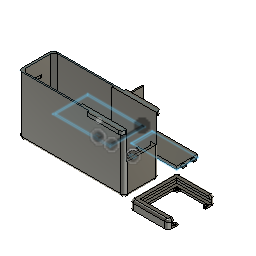
autodoorlock_main_casing v4 (Autodesk Fusion 360 design; units mm, degrees)
Autodesk Fusion 360 part; units mm, degrees
sketch "Sketch1" plane through (0, 0, 0) normal (0, 0, 1) x (1, 0, 0)
  line L0 (-75, 25) -> (75, 25)
  line L1 (75, 25) -> (75, -25)
  line L2 (75, -25) -> (-75, -25)
  line L3 (-75, -25) -> (-75, 25)
  line L4 (16.5, -10.5) -> (58.5, -10.5)
  line L5 (58.5, -10.5) -> (58.5, 10.5)
  line L6 (58.5, 10.5) -> (16.5, 10.5)
  line L7 (16.5, 10.5) -> (16.5, -10.5)
  line L8 (16.5, -10.5) -> (58.5, 10.5) construction
  line L9 (58.5, -10.5) -> (16.5, 10.5) construction
  line L10 (9.5, 10.5) -> (9.5, -10.5065)
  line L11 (16.5, -10.5065) -> (16.5, 10.5)
  line L12 (65.5, 10.5) -> (65.5, -10.5)
  line L13 (58.5, -10.5) -> (58.5, 10.5)
  line L14 (9.5, 10.5) -> (6.5, 10.5)
  line L15 (6.5, 10.5) -> (6.5, -10.5)
  line L16 (6.5, -10.5) -> (9.5, -10.5)
  line L17 (9.5, -10.5) -> (9.5, 10.5)
  line L18 (65.5, 10.5) -> (68.5, 10.5)
  line L19 (68.5, 10.5) -> (68.5, -10.5)
  line L20 (68.5, -10.5) -> (65.5, -10.5)
  line L21 (65.5, -10.5) -> (65.5, 10.5)
  point P0 (37.5, 0)
  dimension "d1" = 150
  dimension "d2" = 50
  dimension "d3" = 42
  dimension "d4" = 21
  dimension "d5" = 7
  dimension "d6" = 7
  dimension "d7" = 21
  dimension "d8" = 3
  dimension "d9" = 21
  dimension "d10" = 3
  dimension "d11" = 21
  constraint horizontal L0
  constraint vertical L1
  constraint horizontal L2
  constraint vertical L3
  constraint horizontal L4
  constraint perpendicular L4 L5
  constraint parallel L4 L6
  constraint parallel L5 L7
  constraint coincident L8 P0
  constraint coincident L9 P0
  constraint vertical L10
  constraint vertical L11
  constraint vertical L12
  constraint vertical L13
  constraint horizontal L14
  constraint vertical L15
  constraint horizontal L16
  constraint vertical L17
  constraint horizontal L18
  constraint vertical L19
  constraint horizontal L20
  constraint vertical L21
  measures "d1" distance of L0.start L0.end
  measures "d2" distance of L0.start L2.end
  measures "d3" distance of L5.end L6.end
  measures "d4" distance of L4.end L5.end
  measures "d5" distance of L6.end L10.start
  measures "d6" distance of L5.end L12.start
  measures "d7" distance of L5.end L4.end
  measures "d8" distance of L10.start L14.end
  measures "d9" distance of L10.start L16.end
  measures "d10" distance of L12.start L18.end
  measures "d11" distance of L12.start L12.end
extrude "Extrude1" add sketch "Sketch1" along normal blind 5 makes body 1
extrude "Extrude2" add sketch "Sketch1" along normal blind 40 contours L10 L14 L15 L16 L17 | L12 L18 L19 L20 L21 bodies 1
sketch "Sketch2" plane through (9.5, 0, 0) normal (1, 0, 0) x (0, 1, 0)
  line L0 (-10.5, 5) -> (10.5, 5)
  line L1 (10.5, 5) -> (10.5, 40)
  line L2 (10.5, 40) -> (-10.5, 40)
  line L3 (-10.5, 40) -> (-10.5, 5)
  line L4 (-10.5, 40) -> (10.5, 40)
  line L5 (10.5, 40) -> (10.5, 35)
  line L6 (10.5, 35) -> (-10.5, 35)
  line L7 (-10.5, 35) -> (-10.5, 40)
  dimension "d16" = 5
  constraint horizontal L4
  constraint vertical L5
  constraint horizontal L6
  constraint vertical L7
  constraint coincident L2.end L3.start
  measures "d16" distance of L2.end L6.end
extrude "Extrude3" add sketch "Sketch2" along normal blind 6 contours L1 L2 L3 L4 L5 L6 L7 bodies 1
sketch "Sketch3" plane through (65.5, 0, 0) normal (-1, 0, 0) x (0, -1, 0)
  line L0 (-10.5, 5) -> (10.5, 5)
  line L1 (10.5, 5) -> (10.5, 40)
  line L2 (10.5, 40) -> (-10.5, 40)
  line L3 (-10.5, 40) -> (-10.5, 5)
  line L4 (-10.5, 40) -> (10.5, 40)
  line L5 (10.5, 40) -> (10.5, 35)
  line L6 (10.5, 35) -> (-10.5, 35)
  line L7 (-10.5, 35) -> (-10.5, 40)
  dimension "d19" = 5
  constraint horizontal L4
  constraint vertical L5
  constraint horizontal L6
  constraint vertical L7
  constraint coincident L2.end L3.start
  measures "d19" distance of L2.end L6.end
extrude "Extrude4" add sketch "Sketch3" along normal blind 6 contours L1 L2 L3 L4 L5 L6 L7 bodies 1
chamfer "Chamfer1" distance 3 angle 45 1 edges at (65.5, 0, 5) on bodies 1
chamfer "Chamfer2" distance 3 angle 45 1 edges at (9.5, 0, 5) on bodies 1
chamfer "Chamfer3" distance 3 angle 45 1 edges at (68.5, 0, 5) on bodies 1
chamfer "Chamfer4" distance 3 angle 45 1 edges at (6.5, 0, 5) on bodies 1
chamfer "Chamfer5" distance 3 angle 45 1 edges at (67, -10.5, 5) on bodies 1
chamfer "Chamfer6" distance 3 angle 45 1 edges at (67, 10.5, 5) on bodies 1
chamfer "Chamfer7" distance 3 angle 45 1 edges at (8, 10.5, 5) on bodies 1
chamfer "Chamfer8" distance 3 angle 45 1 edges at (8, -10.5, 5) on bodies 1
sketch "Sketch4" plane through (0, 0, 40) normal (0, 0, 1) x (-1, 0, 0)
  line L0 (-15.5, -10.5) -> (-6.5, -10.5)
  line L1 (-6.5, -10.5) -> (-6.5, 10.5)
  line L2 (-6.5, 10.5) -> (-15.5, 10.5)
  line L3 (-15.5, 10.5) -> (-15.5, -10.5)
  circle A0 centre (-13.25, 5.25) radius 2.5
  circle A1 centre (-13.25, -5.25) radius 2.5
  dimension "d30" = 5
  dimension "d31" = 5
  measures "d30" diameter of A0
  measures "d31" diameter of A1
extrude "Extrude5" cut sketch "Sketch4" against normal blind 7 contours L3 A1 | L3 A0 picked at (-13.4213, -4.5833) picked at (-12.8787, 5.7617) bodies 1
sketch "Sketch5" plane through (0, 0, 40) normal (0, 0, 1) x (-1, 0, 0)
  line L0 (-59.5, 10.5) -> (-68.5, 10.5)
  line L1 (-68.5, 10.5) -> (-68.5, -10.5)
  line L2 (-68.5, -10.5) -> (-59.5, -10.5)
  line L3 (-59.5, -10.5) -> (-59.5, 10.5)
  circle A0 centre (-61.75, 5.25) radius 2.5
  circle A1 centre (-61.75, -5.25) radius 2.5
  dimension "d34" = 5
  dimension "d35" = 5
  measures "d34" diameter of A0
  measures "d35" diameter of A1
extrude "Extrude6" cut sketch "Sketch5" against normal blind 7 contours L3 A0 | L3 A1 picked at (-61.1713, 5.0046) picked at (-61.1713, -5.4954) bodies 1
extrude "Extrude7" add sketch "Sketch1" along normal blind 5 contours L4 L5 L6 L7 L11 L13 bodies 1
sketch "Sketch6" plane through (0, 0, 35) normal (0, 0, -1) x (1, 0, 0)
  arc A0 (15.5, -4.1603) -> (15.5, -6.3397) centre (13.25, -5.25) ccw
  line L0 (15.5, -4.1603) -> (15.5, 4.1603)
  arc A1 (15.5, 6.3397) -> (15.5, 4.1603) centre (13.25, 5.25) ccw
  line L1 (15.5, 6.3397) -> (15.5, 10.5)
  line L2 (15.5, 10.5) -> (9.5, 10.5)
  line L3 (9.5, 10.5) -> (9.5, -10.5)
  line L4 (9.5, -10.5) -> (15.5, -10.5)
  line L5 (15.5, -10.5) -> (15.5, -6.3397)
  line L6 (15.5, 1.5) -> (9.5, 1.5)
  line L7 (9.5, 1.5) -> (9.5, -1.5)
  line L8 (9.5, -1.5) -> (15.5, -1.5)
  line L9 (15.5, -1.5) -> (15.5, 1.5)
  line L10 (15.5, 1.5) -> (9.5, -1.5) construction
  line L11 (9.5, 1.5) -> (15.5, -1.5) construction
  point P0 (12.5, 0)
  constraint horizontal L6
  constraint perpendicular L6 L7
  constraint parallel L6 L8
  constraint parallel L7 L9
  constraint coincident L10 P0
  constraint coincident L11 P0
  constraint coincident L0 L6.start
delete_face "DeleteFace1" 1 faces at (11.5, -3.5, 6) on bodies 1
delete_face "DeleteFace2" 1 faces at (63.5, -3.5, 6) on bodies 1
sketch "Sketch7" plane through (0, 0, 35) normal (0, 0, -1) x (1, 0, 0)
  arc A0 (59.5, 4.1603) -> (59.5, 6.3397) centre (61.75, 5.25) ccw
  line L0 (59.5, 4.1603) -> (59.5, -4.1603)
  arc A1 (59.5, -6.3397) -> (59.5, -4.1603) centre (61.75, -5.25) ccw
  line L1 (59.5, -6.3397) -> (59.5, -10.5)
  line L2 (59.5, -10.5) -> (65.5, -10.5)
  line L3 (65.5, -10.5) -> (65.5, 10.5)
  line L4 (65.5, 10.5) -> (59.5, 10.5)
  line L5 (59.5, 10.5) -> (59.5, 6.3397)
  line L6 (59.5, 1.5) -> (65.5, 1.5)
  line L7 (65.5, 1.5) -> (65.5, -1.5)
  line L8 (65.5, -1.5) -> (59.5, -1.5)
  line L9 (59.5, -1.5) -> (59.5, 1.5)
  line L10 (59.5, 1.5) -> (65.5, -1.5) construction
  line L11 (65.5, 1.5) -> (59.5, -1.5) construction
  point P0 (62.5, 0)
  dimension "d42" = 3
  constraint horizontal L6
  constraint perpendicular L6 L7
  constraint parallel L6 L8
  constraint parallel L7 L9
  constraint coincident L10 P0
  constraint coincident L11 P0
  measures "d42" distance of L6.end L7.end
extrude "Extrude9" add sketch "Sketch7" along normal blind 30 contours L0 L3 L6 L7 L8 L9 bodies 1
chamfer "Chamfer9" distance 3 angle 45 2 edges at (65.5, 7.5, 5) (62.5, 1.5, 5) on bodies 1
chamfer "Chamfer10" distance 3 angle 45 2 edges at (65.5, -7.5, 5) (62.5, -1.5, 5) on bodies 1
chamfer "Chamfer14" distance 3 angle 45 1 edges at (59.5, 0, 5) on bodies 1
chamfer "Chamfer15" distance 3 angle 45 1 edges at (9.5, 0, 5) on bodies 1
extrude "Extrude10" add sketch "Sketch6" along normal blind 5 contours L0 L3 L6 L7 L8 L9 bodies 1
chamfer "Chamfer16" distance 5 angle 45 1 edges at (15.5, 0, 30) on bodies 1
sketch "Sketch8" plane through (-75, 0, 0) normal (-1, 0, 0) x (0, -1, 0)
  line L0 (-25, 0) -> (25, 0)
  line L1 (25, 0) -> (25, 5)
  line L2 (25, 5) -> (-25, 5)
  line L3 (-25, 5) -> (-25, 0)
  line L4 (-15, 0) -> (15, 0)
  line L5 (15, 0) -> (15, 5)
  line L6 (15, 5) -> (-15, 5)
  line L7 (-15, 5) -> (-15, 0)
  line L8 (-15, 0) -> (15, 5) construction
  line L9 (15, 0) -> (-15, 5) construction
  point P0 (0, 2.5)
  dimension "d55" = 30
  constraint horizontal L4
  constraint perpendicular L4 L5
  constraint parallel L4 L6
  constraint parallel L5 L7
  constraint coincident L8 P0
  constraint coincident L9 P0
  measures "d55" distance of L5.end L6.end
extrude "Extrude11" cut sketch "Sketch8" against normal blind 65 contours L0 L2 L4 L5 L6 L7 bodies 1
sketch "Sketch9" plane through (0, 0, 5) normal (0, 0, 1) x (-1, 0, 0)
  line L0 (10, 15) -> (75, 15)
  line L1 (75, 15) -> (75, 25)
  line L2 (75, 25) -> (-75, 25)
  line L3 (-75, 25) -> (-75, -25)
  line L4 (-75, -25) -> (75, -25)
  line L5 (75, -25) -> (75, -15)
  line L6 (75, -15) -> (10, -15)
  line L7 (10, -15) -> (10, 15)
  line L8 (-12.5, 13.5) -> (-3.5, 13.5)
  line L9 (-3.5, 13.5) -> (-3.5, -13.5)
  line L10 (-3.5, -13.5) -> (-12.5, -13.5)
  line L11 (-12.5, -13.5) -> (-12.5, 13.5)
  line L12 (-56.5, -4.5) -> (-62.5, -4.5)
  line L13 (-62.5, -4.5) -> (-62.5, -13.5)
  line L14 (-62.5, -13.5) -> (-71.5, -13.5)
  line L15 (-71.5, -13.5) -> (-71.5, 13.5)
  line L16 (-71.5, 13.5) -> (-62.5, 13.5)
  line L17 (-62.5, 13.5) -> (-62.5, 4.5)
  line L18 (-62.5, 4.5) -> (-56.5, 4.5)
  line L19 (-56.5, 4.5) -> (-56.5, -4.5)
  line L20 (10, -15) -> (5, -15)
  line L21 (5, -15) -> (5, 15)
  line L22 (5, 15) -> (10, 15)
  line L23 (10, 15) -> (10, -15)
  dimension "d58" = 5
  dimension "d59" = 30
  constraint horizontal L20
  constraint vertical L21
  constraint horizontal L22
  constraint vertical L23
  constraint coincident L6.end L7.start
  measures "d58" distance of L6.end L20.end
  measures "d59" distance of L6.end L0.start
sketch "Sketch10" plane through (0, 0, 5) normal (0, 0, 1) x (-1, 0, 0)
  line L0 (5, 15) -> (75, 15)
  line L1 (75, 15) -> (75, 17)
  line L2 (75, 17) -> (5, 17)
  line L3 (5, 17) -> (5, 15)
  line L4 (5, -15) -> (75, -15)
  line L5 (75, -15) -> (75, -17)
  line L6 (75, -17) -> (5, -17)
  line L7 (5, -17) -> (5, -15)
  point P0 (5, 15)
  point P1 (5, -15)
  dimension "d60" = 2
  dimension "d61" = 2
  constraint horizontal L0
  constraint vertical L1
  constraint horizontal L2
  constraint vertical L3
  constraint coincident P0 L0.start
  constraint horizontal L4
  constraint vertical L5
  constraint horizontal L6
  constraint vertical L7
  constraint coincident P1 L4.start
  measures "d60" distance of P0 L2.end
  measures "d61" distance of P1 L6.end
extrude "Extrude12" add sketch "Sketch10" sketch "Sketch9" along normal blind 20 of sketch 2 contours L7 L20 L21 L22 L23 bodies 1
sketch "Sketch11" plane through (0, 0, 25) normal (0, 0, 1) x (-1, 0, 0)
  line L0 (5, -17) -> (75, -17)
  line L1 (75, -17) -> (75, -15)
  line L2 (75, -15) -> (10, -15)
  line L3 (10, -15) -> (10, 15)
  line L4 (10, 15) -> (75, 15)
  line L5 (75, 15) -> (75, 17)
  line L6 (75, 17) -> (5, 17)
  line L7 (5, 17) -> (5, -17)
  line L8 (5, -17) -> (75, -17)
  line L9 (75, -17) -> (75, 17)
  line L10 (75, 17) -> (5, 17)
  line L11 (5, 17) -> (5, -17)
  constraint horizontal L8
  constraint vertical L9
  constraint horizontal L10
  constraint vertical L11
  constraint coincident L5.end L6.start
  constraint coincident L0.start L7.end
extrude "Extrude13" add sketch "Sketch11" along normal blind 3 bodies 1
sketch "Sketch12" plane through (0, -15, 0) normal (0, 1, 0) x (-1, 0, 0)
  line L0 (75, 0) -> (75, 25)
  line L1 (75, 25) -> (10, 25)
  line L2 (10, 25) -> (10, 0)
  line L3 (10, 0) -> (75, 0)
  line L4 (10, 20.5612) -> (13, 20.5612)
  line L5 (13, 20.5612) -> (13, 5.5612)
  line L6 (13, 5.5612) -> (10, 5.5612)
  line L7 (10, 5.5612) -> (10, 20.5612)
  dimension "d66" = 3
  dimension "d67" = 15
  constraint horizontal L4
  constraint vertical L5
  constraint horizontal L6
  constraint vertical L7
  constraint coincident L2 L4.start
  measures "d66" distance of L4.start L4.end
  measures "d67" distance of L4.start L6.end
extrude "Extrude14" cut sketch "Sketch12" against normal blind 6 contours L2 L4 L5 L6 L7 bodies 1
sketch "Sketch13" plane through (-10, 0, 0) normal (-1, 0, 0) x (0, -1, 0)
  line L0 (-15, 25) -> (-15, 0)
  line L1 (-15, 0) -> (15, 0)
  line L2 (15, 0) -> (15, 5.5612)
  line L3 (15, 5.5612) -> (17, 5.5612)
  line L4 (17, 5.5612) -> (17, 20.5612)
  line L5 (17, 20.5612) -> (15, 20.5612)
  line L6 (15, 20.5612) -> (15, 25)
  line L7 (15, 25) -> (-15, 25)
  line L8 (15, 12.5) -> (15, 0)
  line L9 (15, 0) -> (0, 0)
  line L10 (-15, 12.5) -> (-15, 0)
  line L11 (-15, 0) -> (0, 0)
  line L12 (0, 0) -> (15, 0)
  line L13 (15, 0) -> (15, 12.5)
  line L14 (-10, 0.5625) -> (-5, 0.5625)
  line L15 (-5, 0.5625) -> (-5, 2.5625)
  line L16 (-5, 2.5625) -> (-10, 2.5625)
  line L17 (-10, 2.5625) -> (-10, 0.5625)
  line L18 (-10, 0.5625) -> (-5, 2.5625) construction
  line L19 (-5, 0.5625) -> (-10, 2.5625) construction
  line L20 (5, 0.5625) -> (10, 0.5625)
  line L21 (10, 0.5625) -> (10, 2.5625)
  line L22 (10, 2.5625) -> (5, 2.5625)
  line L23 (5, 2.5625) -> (5, 0.5625)
  line L24 (5, 0.5625) -> (10, 2.5625) construction
  line L25 (10, 0.5625) -> (5, 2.5625) construction
  point P0 (-7.5, 1.5625)
  point P1 (7.5, 1.5625)
  dimension "d73" = 5
  dimension "d74" = 2
  dimension "d75" = 5
  dimension "d76" = 2
  constraint coincident L0.end L1.start
  constraint coincident L1.end L2.start
  constraint vertical L8
  constraint horizontal L9
  constraint vertical L10
  constraint horizontal L11
  constraint horizontal L12
  constraint vertical L13
  constraint horizontal L14
  constraint perpendicular L14 L15
  constraint parallel L14 L16
  constraint parallel L15 L17
  constraint coincident L18 P0
  constraint coincident L19 P0
  constraint horizontal L20
  constraint perpendicular L20 L21
  constraint parallel L20 L22
  constraint parallel L21 L23
  constraint coincident L24 P1
  constraint coincident L25 P1
  measures "d73" distance of L15.end L16.end
  measures "d74" distance of L14.end L15.end
  measures "d75" distance of L21.end L22.end
  measures "d76" distance of L20.end L21.end
extrude "Extrude15" cut sketch "Sketch13" against normal blind 5 contours L14 L15 L16 L17 | L20 L21 L22 L23 bodies 1
sketch "Sketch14" plane through (0, 0, 5) normal (0, 0, 1) x (-1, 0, 0)
  line L0 (-56.5, -4.5) -> (-62.5, -4.5)
  line L1 (-62.5, -4.5) -> (-62.5, -13.5)
  line L2 (-62.5, -13.5) -> (-71.5, -13.5)
  line L3 (-71.5, -13.5) -> (-71.5, 13.5)
  line L4 (-71.5, 13.5) -> (-62.5, 13.5)
  line L5 (-62.5, 13.5) -> (-62.5, 4.5)
  line L6 (-62.5, 4.5) -> (-56.5, 4.5)
  line L7 (-56.5, 4.5) -> (-56.5, -4.5)
  line L8 (-12.5, 13.5) -> (-3.5, 13.5)
  line L9 (-3.5, 13.5) -> (-3.5, -13.5)
  line L10 (-3.5, -13.5) -> (-12.5, -13.5)
  line L11 (-12.5, -13.5) -> (-12.5, 13.5)
  line L12 (75, -17) -> (5, -17)
  line L13 (5, -17) -> (5, 17)
  line L14 (5, 17) -> (75, 17)
  line L15 (75, 17) -> (75, 25)
  line L16 (75, 25) -> (-75, 25)
  line L17 (-75, 25) -> (-75, -25)
  line L18 (-75, -25) -> (75, -25)
  line L19 (75, -25) -> (75, -17)
  line L20 (75, 25) -> (-75, 25)
  line L21 (-75, 25) -> (-75, 23)
  line L22 (-75, 23) -> (75, 23)
  line L23 (75, 23) -> (75, 25)
  line L24 (75, -25) -> (-75, -25)
  line L25 (-75, -25) -> (-75, -23)
  line L26 (-75, -23) -> (75, -23)
  line L27 (75, -23) -> (75, -25)
  line L28 (-75, -23) -> (-73, -23)
  line L29 (-73, -23) -> (-73, 23)
  line L30 (-73, 23) -> (-75, 23)
  line L31 (-75, 23) -> (-75, -23)
  line L32 (75, -23) -> (73, -23)
  line L33 (73, -23) -> (73, -17)
  line L34 (73, -17) -> (75, -17)
  line L35 (75, -17) -> (75, -23)
  line L36 (75, 23) -> (73, 23)
  line L37 (73, 23) -> (73, 17)
  line L38 (73, 17) -> (75, 17)
  line L39 (75, 17) -> (75, 23)
  dimension "d79" = 2
  dimension "d80" = 2
  dimension "d81" = 2
  dimension "d82" = 2
  dimension "d83" = 2
  constraint horizontal L20
  constraint vertical L21
  constraint horizontal L22
  constraint vertical L23
  constraint coincident L15.end L16.start
  constraint horizontal L24
  constraint vertical L25
  constraint horizontal L26
  constraint vertical L27
  constraint coincident L18.end L19.start
  constraint horizontal L28
  constraint vertical L29
  constraint horizontal L30
  constraint vertical L31
  constraint horizontal L32
  constraint vertical L33
  constraint horizontal L34
  constraint vertical L35
  constraint horizontal L36
  constraint vertical L37
  constraint horizontal L38
  constraint vertical L39
  measures "d79" distance of L15.end L22.end
  measures "d80" distance of L18.end L26.end
  measures "d81" distance of L25.end L28.end
  measures "d82" distance of L26.end L32.end
  measures "d83" distance of L22.end L36.end
extrude "Extrude16" add sketch "Sketch14" along normal blind 80 contours L12 L19 L26 L32 L33 L34 L35 | L17 L18 L19 L24 L25 L26 L27 L28 L32 | L17 L22 L26 L28 L29 L30 L31 | L14 L15 L22 L36 L37 L38 L39 | L15 L16 L17 L20 L21 L22 L23 L30 L36 bodies 1
sketch "Sketch15" plane through (0, 0, 28) normal (0, 0, 1) x (-1, 0, 0)
  line L0 (5, 17) -> (5, -17)
  line L1 (5, -17) -> (73, -17)
  line L2 (73, -17) -> (75, -17)
  line L3 (75, -17) -> (75, 17)
  line L4 (75, 17) -> (73, 17)
  line L5 (73, 17) -> (5, 17)
  line L6 (75, -17) -> (73, -17)
  line L7 (73, -17) -> (73, 17)
  line L8 (73, 17) -> (75, 17)
  line L9 (75, 17) -> (75, -17)
  constraint horizontal L6
  constraint vertical L7
  constraint horizontal L8
  constraint vertical L9
  constraint coincident L4.end L5.start
  constraint coincident L2.end L3.start
extrude "Extrude17" add sketch "Sketch15" along normal blind 57 contours L2 L3 L4 L6 L7 L8 L9 bodies 1
sketch "Sketch16" plane through (0, 0, 85) normal (0, 0, 1) x (-1, 0, 0)
  line L0 (73, 23) -> (73, -23)
  line L1 (73, -23) -> (-73, -23)
  line L2 (-73, -23) -> (-73, 23)
  line L3 (-73, 23) -> (73, 23)
  line L4 (75, -25) -> (75, 25)
  line L5 (75, 25) -> (-75, 25)
  line L6 (-75, 25) -> (-75, -25)
  line L7 (-75, -25) -> (75, -25)
  line L8 (-73, 23) -> (-75, 23)
  line L9 (-75, 23) -> (-75, -23)
  line L10 (-75, -23) -> (-73, -23)
  line L11 (-73, -23) -> (-73, 23)
  constraint horizontal L8
  constraint vertical L9
  constraint horizontal L10
  constraint vertical L11
  constraint coincident L6 L9.end
  constraint coincident L2.end L3.start
extrude "Extrude18" cut sketch "Sketch16" against normal blind 40 contours L2 L6 L8 L9 L10 L11 bodies 1
sketch "Sketch17" plane through (0, 0, 0) normal (0, 0, 1) x (1, 0, 0)
  line L0 (75, 50) -> (10.2, 50)
  line L1 (10.2, 50) -> (10.2, 79.8)
  line L2 (10.2, 79.8) -> (75, 79.8)
  line L3 (75, 79.8) -> (75, 50)
  line L4 (10.2, 50) -> (13.2, 50)
  line L5 (13.2, 50) -> (13.2, 79.8)
  line L6 (13.2, 79.8) -> (10.2, 79.8)
  line L7 (10.2, 79.8) -> (10.2, 50)
  dimension "d90" = 64.8
  dimension "d91" = 29.8
  dimension "d92" = 3
  constraint horizontal L0
  constraint vertical L1
  constraint horizontal L2
  constraint vertical L3
  constraint horizontal L4
  constraint vertical L5
  constraint horizontal L6
  constraint vertical L7
  measures "d90" distance of L0.start L0.end
  measures "d91" distance of L0.start L2.end
  measures "d92" distance of L0.end L4.end
extrude "Extrude19" add sketch "Sketch17" along normal blind 4 separate body contours L0 L2 L3 L5 makes body 2
sketch "Sketch18" plane through (0, 0, 25) normal (0, 0, -1) x (1, 0, 0)
  line L0 (-10, 15) -> (-75, 15)
  line L1 (-75, 15) -> (-75, -15)
  line L2 (-75, -15) -> (-10, -15)
  line L3 (-10, -15) -> (-10, 15)
  line L4 (-75, 15) -> (-72, 15)
  line L5 (-72, 15) -> (-72, -15)
  line L6 (-72, -15) -> (-75, -15)
  line L7 (-75, -15) -> (-75, 15)
  dimension "d95" = 3
  constraint horizontal L4
  constraint vertical L5
  constraint horizontal L6
  constraint vertical L7
  constraint coincident L0.end L1.start
  measures "d95" distance of L0.end L4.end
extrude "Extrude20" cut sketch "Sketch18" against normal blind 2 contours L0 L1 L2 L4 L5 L6 L7 bodies 1
extrude "Extrude21" add sketch "Sketch17" along normal blind 27 contours L0 L1 L2 L4 L5 L6 L7 bodies 2
sketch "Sketch19" plane through (75, 0, 0) normal (1, 0, 0) x (0, 1, 0)
  line L0 (50, 0) -> (79.8, 0)
  line L1 (79.8, 0) -> (79.8, 4)
  line L2 (79.8, 4) -> (50, 4)
  line L3 (50, 4) -> (50, 0)
  line L4 (79.8, 2) -> (79.8, 0)
  line L5 (79.8, 0) -> (64.9, 0)
  line L6 (50, 2) -> (50, 0)
  line L7 (50, 0) -> (64.9, 0)
  line L8 (59.95, 2.5) -> (54.95, 2.5)
  line L9 (54.95, 2.5) -> (54.95, 0.5)
  line L10 (54.95, 0.5) -> (59.95, 0.5)
  line L11 (59.95, 0.5) -> (59.95, 2.5)
  line L12 (59.95, 2.5) -> (54.95, 0.5) construction
  line L13 (54.95, 2.5) -> (59.95, 0.5) construction
  line L14 (74.85, 2.5) -> (69.85, 2.5)
  line L15 (69.85, 2.5) -> (69.85, 0.5)
  line L16 (69.85, 0.5) -> (74.85, 0.5)
  line L17 (74.85, 0.5) -> (74.85, 2.5)
  line L18 (74.85, 2.5) -> (69.85, 0.5) construction
  line L19 (69.85, 2.5) -> (74.85, 0.5) construction
  point P0 (57.45, 1.5)
  point P1 (72.35, 1.5)
  dimension "d100" = 5
  dimension "d101" = 2
  dimension "d102" = 5
  dimension "d103" = 2
  constraint coincident L0.start L3.end
  constraint vertical L4
  constraint horizontal L5
  constraint coincident L0.end L1.start
  constraint vertical L6
  constraint horizontal L7
  constraint horizontal L8
  constraint perpendicular L8 L9
  constraint parallel L8 L10
  constraint parallel L9 L11
  constraint coincident L12 P0
  constraint coincident L13 P0
  constraint horizontal L14
  constraint perpendicular L14 L15
  constraint parallel L14 L16
  constraint parallel L15 L17
  constraint coincident L18 P1
  constraint coincident L19 P1
  measures "d100" distance of L9.end L10.end
  measures "d101" distance of L8.end L9.end
  measures "d102" distance of L15.end L16.end
  measures "d103" distance of L14.end L15.end
extrude "Extrude22" add sketch "Sketch19" along normal blind 4 contours L8 L9 L10 L11 | L14 L15 L16 L17 bodies 2
sketch "Sketch20" plane through (0, 0, 5) normal (0, 0, 1) x (-1, 0, 0)
  line L0 (73, -23) -> (73, -17)
  line L1 (73, -17) -> (5, -17)
  line L2 (5, -17) -> (5, 17)
  line L3 (5, 17) -> (73, 17)
  line L4 (73, 17) -> (73, 23)
  line L5 (73, 23) -> (-73, 23)
  line L6 (-73, 23) -> (-73, -23)
  line L7 (-73, -23) -> (73, -23)
  line L8 (-56.5, -4.5) -> (-62.5, -4.5)
  line L9 (-62.5, -4.5) -> (-62.5, -13.5)
  line L10 (-62.5, -13.5) -> (-71.5, -13.5)
  line L11 (-71.5, -13.5) -> (-71.5, 13.5)
  line L12 (-71.5, 13.5) -> (-62.5, 13.5)
  line L13 (-62.5, 13.5) -> (-62.5, 4.5)
  line L14 (-62.5, 4.5) -> (-56.5, 4.5)
  line L15 (-56.5, 4.5) -> (-56.5, -4.5)
  line L16 (-12.5, 13.5) -> (-3.5, 13.5)
  line L17 (-3.5, 13.5) -> (-3.5, -13.5)
  line L18 (-3.5, -13.5) -> (-12.5, -13.5)
  line L19 (-12.5, -13.5) -> (-12.5, 13.5)
  circle A0 centre (-37.5, 13.5) radius 3.5
  circle A1 centre (-37.5, -13.5) radius 3.5
  dimension "d106" = 7
  dimension "d107" = 7
  measures "d106" diameter of A0
  measures "d107" diameter of A1
extrude "Extrude23" cut sketch "Sketch20" against normal blind 5 contours A0 | A1 bodies 1
sketch "Sketch21" plane through (0, 0, 85) normal (0, 0, 1) x (-1, 0, 0)
  line L0 (-75, 23) -> (73, 23)
  line L1 (73, 23) -> (73, -23)
  line L2 (73, -23) -> (-75, -23)
  line L3 (-75, -23) -> (-75, -25)
  line L4 (-75, -25) -> (75, -25)
  line L5 (75, -25) -> (75, 25)
  line L6 (75, 25) -> (-75, 25)
  line L7 (-75, 25) -> (-75, 23)
sketch "Sketch22" plane through (0, 0, 0) normal (0, 0, 1) x (1, 0, 0)
  line L0 (0, 80) -> (-82, 80)
  line L1 (-82, 80) -> (-82, 30)
  line L2 (-82, 30) -> (0, 30)
  line L3 (0, 30) -> (0, 80)
  line L4 (-2, 32.25) -> (-80, 32.25)
  line L5 (-80, 32.25) -> (-80, 77.75)
  line L6 (-80, 77.75) -> (-2, 77.75)
  line L7 (-2, 77.75) -> (-2, 32.25)
  point P0 (-41, 55)
  dimension "d110" = 82
  dimension "d111" = 50
  dimension "d112" = 78
  dimension "d113" = 45.5
  constraint horizontal L0
  constraint vertical L1
  constraint horizontal L2
  constraint vertical L3
  constraint horizontal L4
  constraint perpendicular L4 L5
  constraint parallel L4 L6
  constraint parallel L5 L7
  measures "d110" distance of L0.start L0.end
  measures "d111" distance of L0.start L2.end
  measures "d112" distance of L5.end L6.end
  measures "d113" distance of L4.end L5.end
extrude "Extrude24" add sketch "Sketch22" along normal blind 5 separate body contours L4 L5 L6 L7 makes body 3
extrude "Extrude25" add sketch "Sketch22" along normal blind 2 bodies 3
sketch "Sketch23" plane through (0, 0, 2) normal (0, 0, 1) x (-1, 0, 0)
  line L0 (80, -77.75) -> (2, -77.75)
  line L1 (2, -77.75) -> (2, -32.25)
  line L2 (2, -32.25) -> (80, -32.25)
  line L3 (80, -32.25) -> (80, -77.75)
  line L4 (0, -30) -> (0, -80)
  line L5 (0, -80) -> (82, -80)
  line L6 (82, -80) -> (82, -30)
  line L7 (82, -30) -> (0, -30)
  line L8 (2, -77.75) -> (0, -77.75)
  line L9 (0, -77.75) -> (0, -32.25)
  line L10 (0, -32.25) -> (2, -32.25)
  line L11 (2, -32.25) -> (2, -77.75)
  constraint horizontal L8
  constraint vertical L9
  constraint horizontal L10
  constraint vertical L11
  constraint coincident L4 L9.end
  constraint coincident L0.end L1.start
extrude "Extrude26" add sketch "Sketch23" along normal blind 40 contours L1 L4 L8 L9 L10 L11 bodies 3
sketch "Sketch24" plane through (0, 0, 5) normal (0, 0, 1) x (-1, 0, 0)
  circle A0 centre (-37.5, 13.5) radius 3.5
  circle A1 centre (-37.5, -13.5) radius 3.5
  line L0 (73, -23) -> (73, -17)
  line L1 (73, -17) -> (5, -17)
  line L2 (5, -17) -> (5, 17)
  line L3 (5, 17) -> (73, 17)
  line L4 (73, 17) -> (73, 23)
  line L5 (73, 23) -> (-73, 23)
  line L6 (-73, 23) -> (-73, -23)
  line L7 (-73, -23) -> (73, -23)
  line L8 (-56.5, -4.5) -> (-62.5, -4.5)
  line L9 (-62.5, -4.5) -> (-62.5, -13.5)
  line L10 (-62.5, -13.5) -> (-71.5, -13.5)
  line L11 (-71.5, -13.5) -> (-71.5, 13.5)
  line L12 (-71.5, 13.5) -> (-62.5, 13.5)
  line L13 (-62.5, 13.5) -> (-62.5, 4.5)
  line L14 (-62.5, 4.5) -> (-56.5, 4.5)
  line L15 (-56.5, 4.5) -> (-56.5, -4.5)
  line L16 (-12.5, 13.5) -> (-3.5, 13.5)
  line L17 (-3.5, 13.5) -> (-3.5, -13.5)
  line L18 (-3.5, -13.5) -> (-12.5, -13.5)
  line L19 (-12.5, -13.5) -> (-12.5, 13.5)
  line L20 (-73, -23) -> (-3.5, -23)
  line L21 (-3.5, -23) -> (-3.5, -21)
  line L22 (-3.5, -21) -> (-73, -21)
  line L23 (-73, -21) -> (-73, -23)
  line L24 (-73, 23) -> (-3.5, 23)
  line L25 (-3.5, 23) -> (-3.5, 21)
  line L26 (-3.5, 21) -> (-73, 21)
  line L27 (-73, 21) -> (-73, 23)
  dimension "d120" = 2
  dimension "d121" = 2
  constraint horizontal L20
  constraint vertical L21
  constraint horizontal L22
  constraint vertical L23
  constraint coincident L6.end L7.start
  constraint horizontal L24
  constraint vertical L25
  constraint horizontal L26
  constraint vertical L27
  constraint coincident L5.end L6.start
  measures "d120" distance of L6.end L22.end
  measures "d121" distance of L5.end L26.end
extrude "Extrude27" add sketch "Sketch24" along normal blind 80 contours L6 L7 L20 L21 L22 L23 | L5 L6 L24 L25 L26 L27 bodies 1
extrude "Extrude28" add 2 faces at (73, -22.3333, 58.3333) (73, 21.6667, 58.3333) along direction (1, 0, 0) blind 2 on bodies 1 bodies 1
sketch "Sketch25" plane through (0, 0, 5) normal (0, 0, 1) x (-1, 0, 0)
  line L0 (-3.5, -21) -> (-3.5, -23)
  line L1 (-3.5, -23) -> (73, -23)
  line L2 (73, -23) -> (73, -17)
  line L3 (73, -17) -> (5, -17)
  line L4 (5, -17) -> (5, 17)
  line L5 (5, 17) -> (73, 17)
  line L6 (73, 17) -> (73, 23)
  line L7 (73, 23) -> (-3.5, 23)
  line L8 (-3.5, 23) -> (-3.5, 21)
  line L9 (-3.5, 21) -> (-73, 21)
  line L10 (-73, 21) -> (-73, -21)
  line L11 (-73, -21) -> (-3.5, -21)
  line L12 (-12.5, 13.5) -> (-3.5, 13.5)
  line L13 (-3.5, 13.5) -> (-3.5, -13.5)
  line L14 (-3.5, -13.5) -> (-12.5, -13.5)
  line L15 (-12.5, -13.5) -> (-12.5, 13.5)
  line L16 (-56.5, -4.5) -> (-62.5, -4.5)
  line L17 (-62.5, -4.5) -> (-62.5, -13.5)
  line L18 (-62.5, -13.5) -> (-71.5, -13.5)
  line L19 (-71.5, -13.5) -> (-71.5, 13.5)
  line L20 (-71.5, 13.5) -> (-62.5, 13.5)
  line L21 (-62.5, 13.5) -> (-62.5, 4.5)
  line L22 (-62.5, 4.5) -> (-56.5, 4.5)
  line L23 (-56.5, 4.5) -> (-56.5, -4.5)
  circle A0 centre (-37.5, -13.5) radius 3.5
  circle A1 centre (-37.5, 13.5) radius 3.5
  line L24 (-73, -21) -> (-71.5, -21)
  line L25 (-71.5, -21) -> (-71.5, 21)
  line L26 (-71.5, 21) -> (-73, 21)
  line L27 (-73, 21) -> (-73, -21)
  constraint horizontal L24
  constraint vertical L25
  constraint horizontal L26
  constraint vertical L27
  constraint coincident L9 L25.end
  constraint coincident L10.end L11.start
extrude "Extrude29" add sketch "Sketch25" along normal blind 40 contours L9 L10 L11 L19 L24 L25 L26 L27 bodies 1
extrude "Extrude30" add 1 faces at (-1.3333, 62.5833, 42) along direction (0, 0, 1) blind 10 on bodies 3 bodies 3
sketch "Sketch26" plane through (0, 0, 5) normal (0, 0, 1) x (-1, 0, 0)
  line L0 (2, -77.75) -> (80, -77.75)
  line L1 (80, -77.75) -> (80, -32.25)
  line L2 (80, -32.25) -> (2, -32.25)
  line L3 (2, -32.25) -> (2, -77.75)
  line L4 (80, -60) -> (78, -60)
  line L5 (78, -60) -> (78, -50)
  line L6 (78, -50) -> (80, -50)
  line L7 (80, -50) -> (80, -60)
  dimension "d130" = 2
  constraint horizontal L4
  constraint vertical L5
  constraint horizontal L6
  constraint vertical L7
  constraint coincident L1 L4.start
  measures "d130" distance of L4.start L4.end
extrude "Extrude31" add sketch "Sketch26" along normal blind 20 contours L1 L4 L5 L6 L7 bodies 3
sketch "Sketch27" plane through (-80, 0, 0) normal (-1, 0, 0) x (0, -1, 0)
  line L0 (-77.75, 2) -> (-32.25, 2)
  line L1 (-32.25, 2) -> (-32.25, 5)
  line L2 (-32.25, 5) -> (-50, 5)
  line L3 (-50, 5) -> (-50, 25)
  line L4 (-50, 25) -> (-60, 25)
  line L5 (-60, 25) -> (-60, 5)
  line L6 (-60, 5) -> (-77.75, 5)
  line L7 (-77.75, 5) -> (-77.75, 2)
  line L8 (-50, 25) -> (-60, 25)
  line L9 (-60, 25) -> (-60, 22)
  line L10 (-60, 22) -> (-50, 22)
  line L11 (-50, 22) -> (-50, 25)
  dimension "d133" = 3
  constraint horizontal L8
  constraint vertical L9
  constraint horizontal L10
  constraint vertical L11
  constraint coincident L3.end L4.start
  measures "d133" distance of L3.end L10.end
extrude "Extrude32" add sketch "Sketch27" along normal blind 1 contours L3 L4 L5 L8 L9 L10 L11 bodies 3
fillet "Fillet1" radius 0.5 1 edges at (-81, 55, 22) on bodies 3
sketch "Sketch28" plane through (-73, 0, 0) normal (1, 0, 0) x (0, 1, 0)
  line L0 (17, 5) -> (23, 5)
  line L1 (23, 5) -> (23, 85)
  line L2 (23, 85) -> (-23, 85)
  line L3 (-23, 85) -> (-23, 5)
  line L4 (-23, 5) -> (-17, 5)
  line L5 (-17, 5) -> (-17, 28)
  line L6 (-17, 28) -> (17, 28)
  line L7 (17, 28) -> (17, 5)
  line L8 (-5, 85) -> (5, 85)
  line L9 (-5, 66) -> (5, 66)
  line L10 (5, 66) -> (5, 62)
  line L11 (5, 62) -> (-5, 62)
  line L12 (-5, 62) -> (-5, 66)
  dimension "d138" = 4
  constraint horizontal L8
  constraint coincident L2 L8.start
  constraint horizontal L9
  constraint vertical L10
  constraint horizontal L11
  constraint vertical L12
  measures "d138" distance of L9.start L11.end
extrude "Extrude33" cut sketch "Sketch28" against normal blind 1 contours L9 L10 L11 L12 bodies 1
extrude "Extrude34" cut 2 faces at (3.5, 22.3333, 58.3333) (3.5, -22.3333, 58.3333) along direction (1, 0, 0) blind 8 on bodies 1 bodies 1
extrude "Extrude35" cut 2 faces at (-8.3333, 6.6667, 2.5625) (-8.3333, -8.3333, 2.5625) along direction (0, 0, 1) blind 0.3 on bodies 1 bodies 1
extrude "Extrude36" cut 1 faces at (-8.3333, 10, 2.0958) along direction (0, 1, 0) blind 0.1 on bodies 1 bodies 1
extrude "Extrude37" cut 1 faces at (-8.3333, 5, 1.3292) along direction (0, -1, 0) blind 0.1 on bodies 1 bodies 1
extrude "Extrude38" cut 1 faces at (-8.3333, -10, 1.3292) along direction (0, -1, 0) blind 0.1 on bodies 1 bodies 1
extrude "Extrude39" cut 1 faces at (-8.3333, -5, 2.0958) along direction (0, 1, 0) blind 0.1 on bodies 1 bodies 1
extrude "Extrude40" cut 2 faces at (76.3333, 71.5167, 0.5) (76.3333, 56.6167, 0.5) along direction (0, 0, 1) blind 0.2 on bodies 2 bodies 2
extrude "Extrude41" add 2 faces at (76.3333, 73.1833, 2.5) (76.3333, 58.2833, 2.5) along direction (0, 0, 1) blind 0.2 on bodies 2 bodies 2
extrude "Extrude42" add 5 faces at (-75, 19.6667, 58.3333) (-75, 5, 65.6667) (-75, -22.3333, 58.3333) (-75, -19, 1.6667) (-75, 19, 1.6667) along direction (-1, 0, 0) blind 1 on bodies 1 bodies 1
extrude "Extrude43" add 1 faces at (10.2, 59.9333, 9) along direction (-1, 0, 0) blind 1 on bodies 2 bodies 2
sketch "Sketch29" plane through (0, -25, 0) normal (0, -1, 0) x (1, 0, 0)
  line L0 (-76, 0) -> (75, 0)
  line L1 (75, 0) -> (75, 85)
  line L2 (75, 85) -> (-76, 85)
  line L3 (-76, 85) -> (-76, 0)
  line L4 (75, 85) -> (25, 85)
  line L5 (25, 85) -> (25, 80)
  line L6 (25, 80) -> (75, 80)
  line L7 (75, 80) -> (75, 85)
  dimension "d161" = 50
  dimension "d162" = 5
  constraint horizontal L4
  constraint vertical L5
  constraint horizontal L6
  constraint vertical L7
  constraint coincident L1.end L2.start
  measures "d161" distance of L1.end L4.end
  measures "d162" distance of L1.end L6.end
extrude "Extrude44" add sketch "Sketch29" along normal blind 3 contours L1 L2 L4 L5 L6 L7 bodies 1
sketch "Sketch30" plane through (0, 25, 0) normal (0, 1, 0) x (-1, 0, 0)
  line L0 (-75, 0) -> (76, 0)
  line L1 (76, 0) -> (76, 85)
  line L2 (76, 85) -> (-75, 85)
  line L3 (-75, 85) -> (-75, 0)
  line L4 (-75, 85) -> (-25, 85)
  line L5 (-25, 85) -> (-25, 80)
  line L6 (-25, 80) -> (-75, 80)
  line L7 (-75, 80) -> (-75, 85)
  dimension "d165" = 50
  dimension "d166" = 5
  constraint horizontal L4
  constraint vertical L5
  constraint horizontal L6
  constraint vertical L7
  constraint coincident L2.end L3.start
  measures "d165" distance of L2.end L4.end
  measures "d166" distance of L2.end L6.end
extrude "Extrude45" add sketch "Sketch30" along normal blind 3 contours L2 L3 L4 L5 L6 L7 bodies 1
sketch "Sketch31" plane through (0, 0, 0) normal (0, 0, 1) x (1, 0, 0)
  line L0 (150, 30) -> (150, -27)
  line L1 (150, 30) -> (100, 30)
  line L2 (150, -27) -> (100, -27)
  line L3 (100, -27) -> (100, -32)
  line L4 (100, -32) -> (155, -32)
  line L5 (155, -32) -> (155, 35)
  line L6 (155, 35) -> (100, 35)
  line L7 (100, 35) -> (100, 30)
  dimension "d169" = 57
  dimension "d170" = 50
  dimension "d171" = 5
  dimension "d172" = 55
  dimension "d173" = 67
  constraint vertical L0
  constraint perpendicular L0 L1
  constraint perpendicular L0 L2
  constraint perpendicular L2 L3
  constraint perpendicular L3 L4
  constraint perpendicular L4 L5
  constraint perpendicular L5 L6
  constraint perpendicular L1 L7
  measures "d169" distance of L0.start L0.end
  measures "d170" distance of L0.start L1.end
  measures "d171" distance of L2.end L3.end
  measures "d172" distance of L3.end L4.end
  measures "d173" distance of L4.end L5.end
extrude "Extrude46" add sketch "Sketch31" along normal blind 6 separate body makes body 4
sketch "Sketch32" plane through (0, 0, 6) normal (0, 0, 1) x (-1, 0, 0)
  line L0 (-150, -30) -> (-150, 27)
  line L1 (-150, 27) -> (-100, 27)
  line L2 (-100, 27) -> (-100, 32)
  line L3 (-100, 32) -> (-155, 32)
  line L4 (-155, 32) -> (-155, -35)
  line L5 (-155, -35) -> (-100, -35)
  line L6 (-100, -35) -> (-100, -30)
  line L7 (-100, -30) -> (-150, -30)
  line L8 (-100, -35) -> (-155, -35)
  line L9 (-155, -35) -> (-155, -26)
  line L10 (-155, -26) -> (-100, -26)
  line L11 (-100, -26) -> (-100, -35)
  line L12 (-155, -35) -> (-146, -35)
  line L13 (-146, -35) -> (-146, 32)
  line L14 (-146, 32) -> (-155, 32)
  line L15 (-155, 32) -> (-155, -35)
  line L16 (-155, 32) -> (-100, 32)
  line L17 (-100, 32) -> (-100, 23)
  line L18 (-100, 23) -> (-155, 23)
  line L19 (-155, 23) -> (-155, 32)
  dimension "d176" = 9
  dimension "d177" = 9
  dimension "d178" = 9
  constraint horizontal L8
  constraint vertical L9
  constraint horizontal L10
  constraint vertical L11
  constraint coincident L5.end L6.start
  constraint horizontal L12
  constraint vertical L13
  constraint horizontal L14
  constraint vertical L15
  constraint coincident L4.end L5.start
  constraint horizontal L16
  constraint vertical L17
  constraint horizontal L18
  constraint vertical L19
  measures "d176" distance of L5.end L10.end
  measures "d177" distance of L4.end L12.end
  measures "d178" distance of L3.end L18.end
extrude "Extrude47" add sketch "Sketch32" along normal blind 3 bodies 4
move_body "Move1" bodies 4 to x (-1, 0, 0) y (0, 1, 0) z (0, 0, -1) at (245, 0, 0)
sketch "Sketch33" plane through (0, 0, 0) normal (0, 0, 1) x (-1, 0, 0)
  line L0 (-95, 27) -> (-95, -30)
  line L1 (-95, -30) -> (-145, -30)
  line L2 (-145, -30) -> (-145, -35)
  line L3 (-145, -35) -> (-90, -35)
  line L4 (-90, -35) -> (-90, 32)
  line L5 (-90, 32) -> (-145, 32)
  line L6 (-145, 32) -> (-145, 27)
  line L7 (-145, 27) -> (-95, 27)
  line L8 (-90, -35) -> (-145, -35)
  line L9 (-145, -35) -> (-145, -27.5)
  line L10 (-145, -27.5) -> (-90, -27.5)
  line L11 (-90, -27.5) -> (-90, -35)
  line L12 (-90, -35) -> (-97.5, -35)
  line L13 (-97.5, -35) -> (-97.5, 32)
  line L14 (-97.5, 32) -> (-90, 32)
  line L15 (-90, 32) -> (-90, -35)
  line L16 (-90, 32) -> (-145, 32)
  line L17 (-145, 32) -> (-145, 24.5)
  line L18 (-145, 24.5) -> (-90, 24.5)
  line L19 (-90, 24.5) -> (-90, 32)
  dimension "d181" = 7.5
  dimension "d182" = 7.5
  dimension "d183" = 7.5
  constraint horizontal L8
  constraint vertical L9
  constraint horizontal L10
  constraint vertical L11
  constraint coincident L3.end L4.start
  constraint horizontal L12
  constraint vertical L13
  constraint horizontal L14
  constraint vertical L15
  constraint horizontal L16
  constraint vertical L17
  constraint horizontal L18
  constraint vertical L19
  constraint coincident L4.end L5.start
  measures "d181" distance of L3.end L10.end
  measures "d182" distance of L3.end L12.end
  measures "d183" distance of L4.end L18.end
extrude "Extrude48" add sketch "Sketch33" along normal blind 3 bodies 4
sketch "Sketch34" plane through (0, 0, 0) normal (0, 1, 0) x (1, 0, 0)
sketch "Sketch35" plane through (0, 0, 0) normal (0, 1, 0) x (1, 0, 0)
sketch "Sketch36" plane through (0, 0, 0) normal (0, 0, 1) x (1, 0, 0)
move_body "Move2" bodies 4 to x (1, 0, 0) y (0, 1, 0) z (0, 0, 1) at (0, 0, 9)
sketch "Sketch37" plane through (0, 0, 0) normal (0, 0, 1) x (1, 0, 0)
  line L0 (99, 26) -> (104, 26)
  line L1 (104, 26) -> (104, 21)
  line L2 (104, 21) -> (99, 21)
  line L3 (99, 21) -> (99, 26)
  line L4 (145, 26) -> (140, 26)
  line L5 (140, 26) -> (140, 21)
  line L6 (140, 21) -> (145, 21)
  line L7 (145, 21) -> (145, 26)
  line L8 (99, -23) -> (104, -23)
  line L9 (104, -23) -> (104, -18)
  line L10 (104, -18) -> (99, -18)
  line L11 (99, -18) -> (99, -23)
  line L12 (145, -23) -> (140, -23)
  line L13 (140, -23) -> (140, -18)
  line L14 (140, -18) -> (145, -18)
  line L15 (145, -18) -> (145, -23)
  circle A0 centre (142.5, -20.5) radius 1.5
  circle A1 centre (101.5, -20.5) radius 1.5
  circle A2 centre (101.5, 23.5) radius 1.5
  circle A3 centre (142.5, 23.5) radius 1.5
  dimension "d186" = 5
  dimension "d187" = 5
  dimension "d188" = 5
  dimension "d189" = 5
  dimension "d190" = 5
  dimension "d191" = 5
  dimension "d192" = 5
  dimension "d193" = 5
  dimension "d194" = 3
  dimension "d195" = 3
  dimension "d196" = 3
  dimension "d197" = 3
  constraint horizontal L0
  constraint vertical L1
  constraint horizontal L2
  constraint vertical L3
  constraint horizontal L4
  constraint vertical L5
  constraint horizontal L6
  constraint vertical L7
  constraint horizontal L8
  constraint vertical L9
  constraint horizontal L10
  constraint vertical L11
  constraint horizontal L12
  constraint vertical L13
  constraint horizontal L14
  constraint vertical L15
  measures "d186" distance of L0.start L0.end
  measures "d187" distance of L0.start L2.end
  measures "d188" distance of L4.start L4.end
  measures "d189" distance of L4.start L6.end
  measures "d190" distance of L8.start L8.end
  measures "d191" distance of L8.start L10.end
  measures "d192" distance of L12.start L12.end
  measures "d193" distance of L12.start L14.end
  measures "d194" diameter of A0
  measures "d195" diameter of A1
  measures "d196" diameter of A2
  measures "d197" diameter of A3
extrude "Extrude49" add sketch "Sketch37" along normal blind 2 bodies 4
fillet "Fillet2" radius 3 1 edges at (104, 21, 1) on bodies 4
fillet "Fillet3" radius 3 1 edges at (140, 21, 1) on bodies 4
fillet "Fillet4" radius 3 1 edges at (104, -18, 1) on bodies 4
fillet "Fillet5" radius 3 1 edges at (140, -18, 1) on bodies 4
fillet "Fillet6" radius 5 1 edges at (-76, -25, 42.5) on bodies 1
fillet "Fillet7" radius 5 1 edges at (-76, 25, 42.5) on bodies 1
fillet "Fillet8" radius 5 1 edges at (75, -25, 40) on bodies 1
fillet "Fillet9" radius 5 1 edges at (75, 25, 40) on bodies 1
fillet "Fillet10" radius 5 1 edges at (75, -28, 82.5) on bodies 1
fillet "Fillet11" radius 5 1 edges at (75, 28, 82.5) on bodies 1
fillet "Fillet12" radius 5 9 edges at (-76, 17.5, 0) (-74.5355, 23.5355, 0) (-0.5, 25, 0) (73.5355, 23.5355, 0) (75, 0, 0) (73.5355, -23.5355, 0) (-0.5, -25, 0) (-74.5355, -23.5355, 0) (-76, -17.5, 0) on bodies 1
fillet "Fillet13" radius 5 1 edges at (9.2, 64.9, 0) on bodies 2
fillet "Fillet14" radius 5 4 edges at (145, 35, 6) (90, 35, 6) (145, -32, 6) (90, -32, 6) on bodies 4
fillet "Fillet15" radius 3 9 edges at (145, 28.75, 12) (143.5355, 33.5355, 12) (117.5, 35, 12) (91.4645, 33.5355, 12) (90, 1.5, 12) (91.4645, -30.5355, 12) (117.5, -32, 12) (143.5355, -30.5355, 12) (145, -25.75, 12) on bodies 4
chamfer "Chamfer17" distance 5 angle 45 1 edges at (-73, 23, 45) on bodies 1
chamfer "Chamfer18" distance 5 angle 45 1 edges at (-73, -23, 45) on bodies 1
chamfer "Chamfer19" distance 5 angle 45 1 edges at (-80, 32.25, 3.5) on bodies 3
chamfer "Chamfer20" distance 5 angle 45 1 edges at (-80, 77.75, 3.5) on bodies 3
chamfer "Chamfer21" distance 5 angle 45 1 edges at (71.5, -21, 25) on bodies 1
chamfer "Chamfer22" distance 5 angle 45 1 edges at (71.5, 21, 25) on bodies 1
